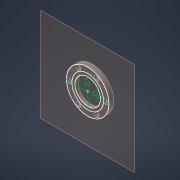
# Autodesk Inventor part: Brida de rodamientos
Saved by Autodesk Inventor 2022 (Build 260153000, 153)
## iProperties
Created: 2021-09-15
Part Number: Brida de rodamientos
Material: Steel, Mild, Welded
Document SubType Name: Modeling
Designer: Andres
Density: 7.85 g/cm^3
Appearance: Weld - Steel Mild
Author: Andres
Autodesk Inventor part; units mm, degrees
ref_plane "YZ Plane" through (0, 0, 0) normal (1, 0, 0) x (0, 1, 0)
ref_plane "XZ Plane" through (0, 0, 0) normal (0, 1, 0) x (-1, 0, 0)
ref_plane "XY Plane" through (0, 0, 0) normal (0, 0, 1) x (1, 0, 0)
ref_plane "Work Plane1" through (0, 0, 0) normal (0, 0, 1) x (1, 0, 0)
sketch "Sketch1" plane through (0, 0, 0) normal (0, 0, 1) x (1, 0, 0)
  circle A0 centre (0, 0) radius 26
  circle A1 centre (0, 0) radius 40
  circle A2 centre (0, 0) radius 21
  dimension "d0" = 52
  dimension "d1" = 80
  dimension "d4" = 42
  constraints: 3 centre point, 3 coincident
  measures "d0" diameter of A0
  measures "d1" diameter of A1
  measures "d4" diameter of A2
extrude "Extrusion1" add sketch "Sketch1" against normal blind 5.5 contours A0
extrude "Extrusion2" add sketch "Sketch1" against normal blind 8 contours A1
sketch "Sketch2" plane through (0, 0, 0) normal (0, 0, 1) x (1, 0, 0)
  circle A0 centre (0, 0) radius 32.5 construction
  point P0 (-32.5, 0)
  point P1 (-16.25, -28.1458)
  point P2 (16.25, -28.1458)
  point P3 (32.5, 0)
  point P4 (16.25, 28.1458)
  point P5 (-16.25, 28.1458)
  dimension "d7" = 65
  dimension "d10" = 360
  constraints: 2 horizontal alignment, 1 coincident, 9 other
hole "Hole1" at (-32.5, 0, 0) at (-16.25, -28.1458, 0) at (16.25, -28.1458, 0) at (32.5, 0, 0) at (16.25, 28.1458, 0) at (-16.25, 28.1458, 0) direction (0, 0, -1) diameter 4.5 depth 8 tip angle 118 counterbore diameter 8 counterbore depth 4.6 clearance for "Socket Head Cap Screw ISO 4762" size "M4" standard "ISO"
body "Solid1"
